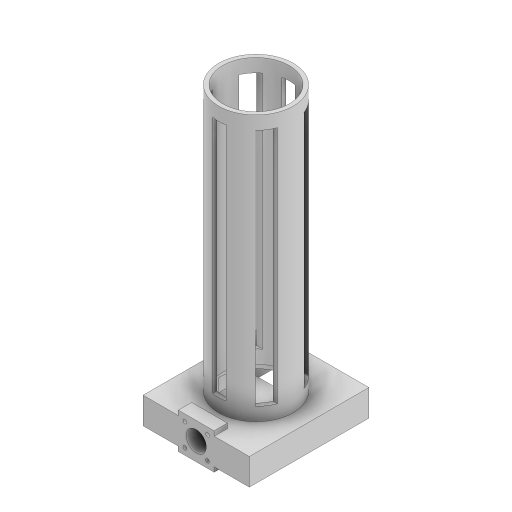
# Autodesk Inventor part: TUBO CONTENEDOR
Saved by Autodesk Inventor 2024 (Build 280153000, 153)
## iProperties
Created: 2024-06-30
Part Number: TUBO CONTENEDOR
Material: Generic
Document SubType Name: Modeling
Designer: Jhuliams
Density: 1 g/cm^3
Appearance: Default
Author: Jhuliams
Autodesk Inventor part; units mm, degrees
ref_plane "YZ Plane" through (0, 0, 0) normal (1, 0, 0) x (0, 1, 0)
ref_plane "XZ Plane" through (0, 0, 0) normal (0, 1, 0) x (-1, 0, 0)
ref_plane "XY Plane" through (0, 0, 0) normal (0, 0, 1) x (1, 0, 0)
sketch "Sketch1" plane through (0, 0, 0) normal (0, 1, 0) x (-1, 0, 0)
  circle A0 centre (0, 0) radius 25
  circle A1 centre (0, 0) radius 28
  dimension "d0" = 50
  dimension "d1" = 56
  constraints: 2 centre point, 2 coincident
  measures "d0" diameter of A0
  measures "d1" diameter of A1
extrude "Extrusion1" add sketch "Sketch1" along normal blind 200
sketch "Sketch2" plane through (0, 0, 0) normal (1, 0, 0) x (0, 1, 0)
  line L0 (0, 0) -> (0, 15)
  line L1 (0, -28) -> (0, 28) projected
  line L2 (0, 15) -> (100, 15)
  line L3 (190, 20) -> (10, 20)
  line L4 (10, 20) -> (10, 10)
  line L5 (10, 10) -> (190, 10)
  line L6 (190, 10) -> (190, 20)
  line L7 (190, 20) -> (10, 10) construction
  line L8 (10, 20) -> (190, 10) construction
  line L9 (0, 0) -> (25, 0)
  line L10 (190, -20) -> (10, -20)
  line L11 (10, -20) -> (10, -10)
  line L12 (10, -10) -> (190, -10)
  line L13 (190, -10) -> (190, -20)
  line L14 (190, -20) -> (10, -10) construction
  line L15 (10, -20) -> (190, -10) construction
  point P0 (100, -15)
  dimension "d4" = 15
  dimension "d5" = 100
  dimension "d6" = 180
  dimension "d7" = 10
  dimension "d8" = 25
  constraints: 30 end point, 5 symmetric about line, 3 horizontal, 2 midpoint, 2 parallel, 1 perpendicular, 1 point on line
  measures "d4" distance of L0.start L0.end
  measures "d5" distance of L0.end L2.end
  measures "d6" distance of L5.end L4.end
  measures "d7" distance of L4.end L3.end
  measures "d8" distance of L0.start L9.end
extrude "Extrusion2" cut sketch "Sketch2" along normal mid plane 100
sketch "Sketch4" plane through (0, 0, 0) normal (0, 0, 1) x (1, 0, 0)
  line L0 (0, 0) -> (0, 100)
  line L1 (-5, 190) -> (5, 190)
  line L2 (5, 190) -> (5, 10)
  line L3 (5, 10) -> (-5, 10)
  line L4 (-5, 10) -> (-5, 190)
  line L5 (-5, 190) -> (5, 10) construction
  line L6 (5, 190) -> (-5, 10) construction
  dimension "d11" = 100
  dimension "d12" = 10
  dimension "d13" = 180
  constraints: 14 end point, 2 midpoint, 2 parallel, 1 horizontal, 1 perpendicular, 1 vertical
  measures "d11" distance of L0.start L0.end
  measures "d12" distance of L2.end L3.end
  measures "d13" distance of L1.end L2.end
extrude "Extrusion3" cut sketch "Sketch4" along normal mid plane 100
sketch "Sketch5" plane through (0, 0, 0) normal (0, -1, 0) x (1, 0, 0)
  line L0 (-40, 45) -> (40, 45)
  line L1 (40, 45) -> (40, -45)
  line L2 (40, -45) -> (-40, -45)
  line L3 (-40, -45) -> (-40, 45)
  line L4 (-40, 45) -> (40, -45) construction
  line L5 (40, 45) -> (-40, -45) construction
  circle A0 centre (0, 0) radius 28
  dimension "d16" = 80
  dimension "d17" = 90
  dimension "d18" = 56
  constraints: 12 end point, 2 midpoint, 2 parallel, 1 centre point, 1 coincident, 1 horizontal, 1 perpendicular
  measures "d16" distance of L1.end L2.end
  measures "d17" distance of L0.end L1.end
  measures "d18" diameter of A0
extrude "Extrusion4" add sketch "Sketch5" along normal blind 20
sketch "Sketch6" plane through (-40, 0, 45) normal (0, 0, 1) x (1, 0, 0)
  circle A0 centre (40, -10) radius 7.6
  point P0 (40, 0)
  dimension "d21" = 15.2
  constraints: 1 centre point
  measures "d21" diameter of A0
extrude "Extrusion5" cut sketch "Sketch6" against normal blind 20
sketch "Sketch7" plane through (0, -20, 0) normal (0, -1, 0) x (1, 0, 0)
  circle A0 centre (0, 0) radius 28 projected
extrude "Extrusion6" add sketch "Sketch7" against normal blind 5
sketch "Sketch8" plane through (40, 0, -45) normal (0, 0, -1) x (-1, 0, 0)
  line L0 (12, 0) -> (12, 200) projected
  line L1 (68, 0) -> (68, 200) projected
  line L2 (80, 0) -> (0, 0) projected
  line L3 (40, 0) -> (40, -10)
  line L4 (12, -15) -> (68, -15) projected
  line L5 (12, -5) -> (68, -5)
  line L6 (68, -5) -> (68, -15)
  line L7 (68, -15) -> (12, -15)
  line L8 (12, -15) -> (12, -5)
  circle A0 centre (40, -10) radius 7.6 projected
  line L9 (12, -5) -> (68, -15) construction
  line L10 (68, -5) -> (12, -15) construction
  point P0 (45.7236, -15)
  point P1 (34.2764, -15)
  dimension "d26" = 10
  constraints: 14 end point, 2 midpoint, 2 parallel, 1 horizontal, 1 perpendicular, 1 vertical
  measures "d26" distance of L3.start L3.end
extrude "Extrusion7" cut sketch "Sketch8" against normal blind 45 contours L5 A0 L4 | L5 L6 L4 A0 | A0 L4 L8 L5
sketch "Sketch9" plane through (-40, 0, 45) normal (0, 0, 1) x (1, 0, 0)
  circle A0 centre (40, -10) radius 7.6 projected
  line L0 (26.5, 3.5) -> (53.5, 3.5)
  line L1 (53.5, 3.5) -> (53.5, -23.5)
  line L2 (53.5, -23.5) -> (26.5, -23.5)
  line L3 (26.5, -23.5) -> (26.5, 3.5)
  line L4 (26.5, 3.5) -> (53.5, -23.5) construction
  line L5 (53.5, 3.5) -> (26.5, -23.5) construction
  circle A1 centre (40, -10) radius 12
  line L6 (53.5, 3.5) -> (26.5, -23.5)
  circle A2 centre (48.4853, -1.5147) radius 1.4
  circle A3 centre (31.5147, -1.5147) radius 1.4
  circle A4 centre (31.5147, -18.4853) radius 1.4
  circle A5 centre (48.4853, -18.4853) radius 1.4
  point P0 (40, 0)
  dimension "d31" = 24
  dimension "d29" = 27
  dimension "d30" = 27
  dimension "d32" = 2.8
  dimension "d39" = 360
  constraints: 14 end point, 4 centre point, 3 equal length, 2 midpoint, 1 coincident, 1 horizontal, 1 perpendicular, 1 point on line, 12 other
  measures "d29" distance of L1.end L2.end
  measures "d30" distance of L0.end L1.end
  measures "d32" diameter of A2
extrude "Extrusion8" add sketch "Sketch9" against normal blind 10 contours A0 L6 A2 A1 A5 A4 | A0 L6 A4 A1 A3 A2 | A1 A3 A4 L6 L3 L0 A2 | A2 L6 L1 L2 A4 A1 A5
extrude "Extrusion9" cut sketch "Sketch9" against normal blind 10 contours A2 A1 L6 | L6 A1 A2 | A4 A1 L6 | L6 A1 A4 | L6 A2 A1 | A1 A2 L6 | L6 A4 A1 | A1 A4 L6 | A3 A1 | A1 A3 | A5 A1 | A1 A5
sketch "Sketch10" plane through (40, 0, -45) normal (0, 0, -1) x (-1, 0, 0)
  line L0 (68, -15) -> (12, -15) projected
  line L1 (53.5, -20) -> (80, -20) projected
  line L2 (12, -10) -> (68, -10)
  line L3 (68, -10) -> (68, -20)
  line L4 (68, -20) -> (12, -20)
  line L5 (12, -20) -> (12, -10)
  line L6 (12, -10) -> (68, -20) construction
  line L7 (68, -10) -> (12, -20) construction
  point P0 (40, 0)
  point P1 (40, -15)
  constraints: 12 end point, 3 midpoint, 2 parallel, 1 horizontal, 1 perpendicular, 1 point on line
extrude "Extrusion10" cut sketch "Sketch10" against normal blind 20
body "Solid1"
